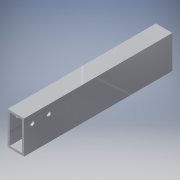
# Autodesk Inventor part: superstructure
Saved by Autodesk Inventor 2016 (Build 200138000, 138)
## iProperties
Created: 2016-01-29
Part Number: superstructure
Material: Aluminum 6061
Document SubType Name: Modeling
Designer: zachary
Density: 2.7 g/cm^3
Appearance: Aluminum - Flat
Mass: 272.54 g
Surface Area: 647.411 cm^2
Volume: 100.941 cm^3
Author: zachary
Autodesk Inventor part; units mm, degrees
ref_plane "YZ Plane" through (0, 0, 0) normal (1, 0, 0) x (0, 1, 0)
ref_plane "XZ Plane" through (0, 0, 0) normal (0, 1, 0) x (-1, 0, 0)
ref_plane "XY Plane" through (0, 0, 0) normal (0, 0, 1) x (1, 0, 0)
sketch "Sketch1" plane through (0, 0, 0) normal (0, 0, 1) x (1, 0, 0)
  line L0 (0, 0) -> (25.4, 0)
  line L1 (25.4, 0) -> (25.4, 50.8)
  line L2 (25.4, 50.8) -> (0, 50.8)
  line L3 (0, 50.8) -> (0, 0)
  line L4 (22.225, 3.175) -> (3.175, 3.175)
  line L5 (3.175, 3.175) -> (3.175, 47.625)
  line L6 (3.175, 47.625) -> (22.225, 47.625)
  line L7 (22.225, 47.625) -> (22.225, 3.175)
  dimension "d0" = 25.4
  dimension "d1" = 50.8
  dimension "d2" = 3.175
  dimension "d3" = 3.175
  dimension "d4" = 3.175
  dimension "d5" = 3.175
  constraints: 16 end point, 4 parallel, 2 horizontal, 2 perpendicular
  measures "d0" distance between parallel lines of L1 L3
  measures "d1" distance between parallel lines of L2 L0
  measures "d2" distance between parallel lines of L5 L3
  measures "d3" distance between parallel lines of L4 L0
  measures "d4" distance between parallel lines of L1 L7
  measures "d5" distance between parallel lines of L2 L6
extrude "Extrusion1" add sketch "Sketch1" along normal blind 228.6
sketch "Sketch2" plane through (0, 0, 0) normal (-1, 0, 0) x (0, 0, 1)
  circle A0 centre (215.9, 38.1) radius 3.3734
  circle A1 centre (190.5, 38.1) radius 3.3734
  line L0 (0, 50.8) -> (228.6, 50.8) projected
  line L1 (228.6, 50.8) -> (228.6, 0) projected
  point P0 (0, 0)
  dimension "d8" = 6.7469
  dimension "d9" = 6.7469
  dimension "d10" = 12.7
  dimension "d11" = 12.7
  dimension "d12" = 12.7
  dimension "d13" = 38.1
  constraints: 2 centre point
  measures "d8" diameter of A0
  measures "d9" diameter of A1
  measures "d10" distance from line of L0 A1.centre
  measures "d11" distance from line of L0 A0.centre
  measures "d12" distance from line of L1 A0.centre
  measures "d13" distance from line of L1 A1.centre
extrude "Extrusion2" cut sketch "Sketch2" against normal blind 25.4
body "Solid1"
